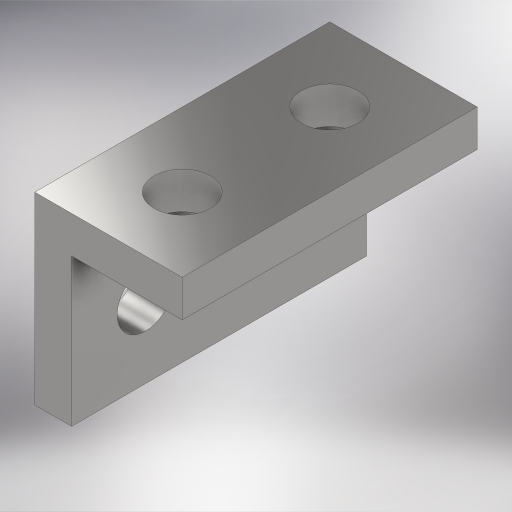
# Autodesk Inventor part: Gusset
Saved by Autodesk Inventor 2024 (Build 280153000, 153)
## iProperties
Created: 2023-11-09
Part Number: Gusset
Material: Stainless Steel
Document SubType Name: Modeling
Designer: aaron
Density: 8 g/cm^3
Appearance: Semi-Polished
Author: aaron
Autodesk Inventor part; units mm, degrees
ref_plane "YZ Plane" through (0, 0, 0) normal (1, 0, 0) x (0, 1, 0)
ref_plane "XZ Plane" through (0, 0, 0) normal (0, 1, 0) x (-1, 0, 0)
ref_plane "XY Plane" through (0, 0, 0) normal (0, 0, 1) x (1, 0, 0)
sketch "Sketch1" plane through (0, 0, 0) normal (0, 0, 1) x (1, 0, 0)
  line L0 (6.35, -7.9375) -> (-6.35, -7.9375)
  line L1 (-6.35, -7.9375) -> (-6.35, 7.9375)
  line L2 (-6.35, 7.9375) -> (6.35, 7.9375)
  line L3 (6.35, 7.9375) -> (6.35, -7.9375)
  line L4 (6.35, -7.9375) -> (-6.35, 7.9375) construction
  line L5 (-6.35, -7.9375) -> (6.35, 7.9375) construction
  line L6 (6.35, -7.9375) -> (-3.175, -7.9375)
  line L7 (-3.175, -7.9375) -> (-3.175, 4.7625)
  line L8 (-3.175, 4.7625) -> (6.35, 4.7625)
  line L9 (6.35, 4.7625) -> (6.35, -7.9375)
  point P0 (0, 0)
  point P1 (-3.175, -7.9375)
  dimension "d0" = 12.7
  dimension "d1" = 15.875
  dimension "d2" = 9.525
  dimension "d3" = 12.7
  constraints: 20 end point, 4 parallel, 2 horizontal, 2 midpoint, 2 perpendicular
  measures "d0" distance of L1.end L2.end
  measures "d1" distance of L0.end L1.end
  measures "d2" distance of L7.end L8.end
  measures "d3" distance of L6.end L7.end
extrude "Extrusion1" add sketch "Sketch1" along normal blind 25.4 contours L0 L1 L2 L3 L8 L7
sketch "Sketch2" plane through (-3.175, 4.7625, 0) normal (0, -1, 0) x (1, 0, 0)
  circle A0 centre (3.175, 19.05) radius 2.4257
  circle A1 centre (3.175, 6.35) radius 2.4257
  line L0 (0, 25.4) -> (9.525, 25.4) projected
  line L1 (0, 0) -> (9.525, 0) projected
  point P0 (3.175, 0)
  point P1 (4.7625, 25.4)
  dimension "d6" = 4.8514
  dimension "d7" = 4.8514
  dimension "d8" = 6.35
  dimension "d9" = 6.35
  constraints: 2 centre point, 1 midpoint
  measures "d6" diameter of A0
  measures "d7" diameter of A1
  measures "d8" vertical distance of point (4.763, 25.4) A0.centre
  measures "d9" distance from line of L1 A1.centre
extrude "Extrusion2" cut sketch "Sketch2" against normal blind 25.4
sketch "Sketch3" plane through (-3.175, -7.9375, 0) normal (1, 0, 0) x (0, 0, -1)
  circle A0 centre (-6.35, 6.35) radius 2.4257
  circle A1 centre (-19.05, 6.35) radius 2.4257
  line L0 (-25.4, 0) -> (-25.4, 12.7) projected
  line L1 (0, 0) -> (0, 12.7) projected
  point P0 (0, 7.9375)
  dimension "d12" = 4.8514
  dimension "d13" = 4.8514
  dimension "d14" = 6.35
  dimension "d15" = 6.35
  constraints: 2 centre point
  measures "d12" diameter of A0
  measures "d13" diameter of A1
  measures "d14" distance from line of L0 A1.centre
  measures "d15" distance from line of A0.centre L1
extrude "Extrusion3" cut sketch "Sketch3" against normal blind 25.4
body "Solid1"
